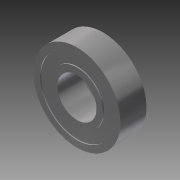
# Autodesk Inventor part: Bearing 699ZZ - 9x20x6mm
Saved by Autodesk Inventor 2013 (Build 170138000, 138)
## iProperties
Created: 2014-10-09
Part Number: Bearing 699ZZ - 9x20x6mm
Material: Stainless Steel
Document SubType Name: Modeling
Designer: Masta
Density: 8.08 g/cm^3
Mass: 11.6862 g
Surface Area: 10.9327 cm^2
Volume: 1.44631 cm^3
Author: Masta
Autodesk Inventor part; units mm, degrees
ref_plane "YZ Plane" through (0, 0, 0) normal (1, 0, 0) x (0, 1, 0)
ref_plane "XZ Plane" through (0, 0, 0) normal (0, 1, 0) x (-1, 0, 0)
ref_plane "XY Plane" through (0, 0, 0) normal (0, 0, 1) x (1, 0, 0)
sketch "Sketch1" plane through (0, 0, 0) normal (0, 1, 0) x (-1, 0, 0)
  circle A0 centre (0, 0) radius 4.5
  circle A1 centre (0, 0) radius 6
  circle A2 centre (0, 0) radius 10
  circle A3 centre (0, 0) radius 8.5
  dimension "d0" = 9
  dimension "d2" = 20
  dimension "d3" = 1.5
  dimension "d4" = 1.5
  constraints: 4 centre point, 4 coincident
  measures "d0" diameter of A0
  measures "d2" diameter of A2
  measures "d3" radial gap between concentric circles of A1 A0
  measures "d4" radial gap between concentric circles of A2 A3
extrude "Extrusion1" add sketch "Sketch1" along normal mid plane 6
extrude "Extrusion2" add sketch "Sketch1" along normal mid plane 5.5 contours A3
body "Solid1"
